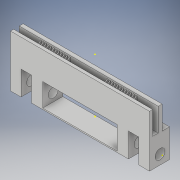
# Autodesk Inventor part: Xbelt Holder
Saved by Autodesk Inventor 2018 (Build 220112000, 112)
## iProperties
Created: 2018-02-26
Part Number: Xbelt Holder
Material: Generic
Document SubType Name: Modeling
Designer: junai
Density: 1 g/cm^3
Appearance: Default
Mass: 48.8128 g
Surface Area: 308.114 cm^2
Volume: 48.8128 cm^3
Author: junai
Autodesk Inventor part; units mm, degrees
ref_plane "YZ Plane" through (0, 0, 0) normal (1, 0, 0) x (0, 1, 0)
ref_plane "XZ Plane" through (0, 0, 0) normal (0, 1, 0) x (-1, 0, 0)
ref_plane "XY Plane" through (0, 0, 0) normal (0, 0, 1) x (1, 0, 0)
sketch "Sketch1" plane through (0, 0, 0) normal (0, 1, 0) x (-1, 0, 0)
  point P0 (0, 0)
sketch "Sketch2" plane through (0, 0, 0) normal (0, 1, 0) x (-1, 0, 0)
  line L0 (68.1059, 14.081) -> (-63.8941, 14.081)
  line L1 (-63.8941, 14.081) -> (-63.8941, -10.919)
  line L2 (-63.8941, -10.919) -> (68.1059, -10.919)
  line L3 (68.1059, -10.919) -> (68.1059, 14.081)
  point P0 (0, 0)
  dimension "d0" = 132
  dimension "d1" = 25
  constraints: 8 end point, 2 parallel, 1 horizontal, 1 perpendicular
  measures "d0" distance of L2.end L1.end
  measures "d1" distance of L0.end L1.end
extrude "Extrusion2" add sketch "Sketch2" along normal blind 6
sketch "Sketch4" plane through (0, 6, 0) normal (0, 1, 0) x (1, 0, 0)
  line L0 (-68.1059, -14.081) -> (63.8941, -14.081) projected
  line L1 (-68.1059, -14.081) -> (63.8941, -14.081)
  line L2 (63.8941, -14.081) -> (63.8941, -9.081)
  line L3 (63.8941, -9.081) -> (-68.1059, -9.081)
  line L4 (-68.1059, -9.081) -> (-68.1059, -14.081)
  line L5 (63.8941, -14.081) -> (63.8941, 10.919) projected
  point P0 (0, 0)
  dimension "d7" = 5
  constraints: 8 end point, 2 parallel, 1 collinear, 1 horizontal, 1 perpendicular
  measures "d7" distance of L1.end L2.end
extrude "Extrusion3" add sketch "Sketch4" along normal blind 45
sketch "Sketch5" plane through (0, 6, 0) normal (0, 1, 0) x (1, 0, 0)
  line L0 (63.8941, 10.919) -> (-68.1059, 10.919) projected
  line L1 (-68.1059, 10.919) -> (63.8941, 10.919)
  line L2 (63.8941, 10.919) -> (63.8941, -1.081)
  line L3 (63.8941, -1.081) -> (-68.1059, -1.081)
  line L4 (-68.1059, -1.081) -> (-68.1059, 10.919)
  line L5 (63.8941, -9.081) -> (63.8941, 10.919) projected
  point P0 (0, 0)
  dimension "d10" = 12
  constraints: 8 end point, 2 parallel, 1 collinear, 1 horizontal, 1 perpendicular
  measures "d10" distance of L1.end L2.end
extrude "Extrusion4" add sketch "Sketch5" along normal blind 45
sketch "Sketch6" plane through (0, 0, 0) normal (0, -1, 0) x (1, 0, 0)
  line L0 (63.8941, -10.919) -> (-68.1059, -10.919) projected
  line L1 (63.8941, -10.919) -> (-68.1059, -10.919)
  line L2 (-68.1059, -10.919) -> (-68.1059, -1.919)
  line L3 (-68.1059, -1.919) -> (63.8941, -1.919)
  line L4 (63.8941, -1.919) -> (63.8941, -10.919)
  line L5 (-68.1059, -10.919) -> (-68.1059, 14.081) projected
  point P0 (0, 0)
  dimension "d13" = 9
  constraints: 8 end point, 2 parallel, 1 collinear, 1 horizontal, 1 perpendicular
  measures "d13" distance of L1.end L2.end
extrude "Extrusion5" cut sketch "Sketch6" against normal blind 26
sketch "Sketch10" plane through (0, 51, 0) normal (0, 1, 0) x (1, 0, 0)
  point P0 (0, 0)
sketch "Sketch11" plane through (0, 51, 0) normal (0, 1, 0) x (1, 0, 0)
  line L0 (-58.1059, 1.919) -> (-48.1059, 1.919) construction
  line L1 (53.8941, 1.919) -> (43.8941, 1.919) construction
  line L2 (63.8941, 10.919) -> (-68.1059, 10.919) projected
  line L3 (-48.1059, 1.919) -> (-58.1059, 1.919)
  line L4 (-58.1059, 1.919) -> (-58.1059, 10.919)
  line L5 (-58.1059, 10.919) -> (-48.1059, 10.919)
  line L6 (-48.1059, 10.919) -> (-48.1059, 1.919)
  line L7 (43.8941, 1.919) -> (53.8941, 1.919)
  line L8 (53.8941, 1.919) -> (53.8941, 10.919)
  line L9 (53.8941, 10.919) -> (43.8941, 10.919)
  line L10 (43.8941, 10.919) -> (43.8941, 1.919)
  line L11 (-68.1059, -1.081) -> (-68.1059, -9.081) construction
  line L12 (-68.1059, -1.081) -> (-58.1059, -1.081) construction
  line L13 (-58.1059, -1.081) -> (-58.1059, 1.919) construction
  line L14 (63.8941, -1.081) -> (53.8941, -1.081) construction
  line L15 (-68.1059, -1.081) -> (63.8941, -1.081) construction
  line L16 (53.8941, -1.081) -> (53.8941, 1.919) construction
  point P0 (0, 0)
  dimension "d21" = 10
  dimension "d23" = 10
  dimension "d26" = 10
  dimension "d27" = 9
  dimension "d28" = 9
  dimension "d29" = 10
  dimension "d30" = 10
  constraints: 28 end point, 4 parallel, 4 perpendicular, 3 horizontal, 3 point on line
  measures "d21" distance of L0.start L0.end
  measures "d23" distance of L1.start L1.end
  measures "d26" distance between parallel lines of L6 L4
  measures "d27" distance of L9.end L1.end
  measures "d28" distance of L5.end L0.end
  measures "d29" distance of L11.start L12.end
  measures "d30" distance of L14.start L14.end
extrude "Extrusion6" cut sketch "Sketch11" against normal blind 26
sketch "Sketch13" plane through (0, 6, 0) normal (0, 1, 0) x (1, 0, 0)
  line L0 (-48.1059, 1.919) -> (-48.1059, -9.1654) construction
  line L1 (-48.1059, -1.081) -> (-47.0059, -1.081)
  constraints: 4 end point, 1 horizontal, 1 point on line, 1 vertical
sketch "Sketch14" plane through (0, 51, 0) normal (0, 1, 0) x (1, 0, 0)
  line L0 (-68.1059, -1.081) -> (-68.1059, -9.081) projected
  line L1 (-68.1059, -1.081) -> (63.8941, -1.081)
  line L2 (63.8941, -1.081) -> (63.8941, -4.081)
  line L3 (63.8941, -4.081) -> (-68.1059, -4.081)
  line L4 (-68.1059, -4.081) -> (-68.1059, -1.081)
  line L5 (63.8941, -9.081) -> (63.8941, -1.081) projected
  point P0 (0, 0)
  dimension "d35" = 3
  constraints: 8 end point, 2 parallel, 1 collinear, 1 horizontal, 1 perpendicular
  measures "d35" distance of L1.end L2.end
extrude "Extrusion7" add sketch "Sketch14" against normal up to next
sketch "Sketch15" plane through (0, 51, 0) normal (0, 1, 0) x (1, 0, 0)
  line L0 (-68.1059, 1.919) -> (63.8941, 1.919) projected
  line L1 (-58.3742, 1.919) -> (-48.1059, 1.919)
  line L2 (-48.1059, 1.919) -> (-48.1059, -0.081)
  line L3 (-48.1059, -0.081) -> (-58.3742, -0.081)
  line L4 (-58.3742, -0.081) -> (-58.3742, 1.919)
  line L5 (-48.1059, 10.919) -> (-48.1059, 1.919) projected
  line L6 (53.8941, 1.919) -> (43.8941, 1.919) projected
  line L7 (43.8941, 1.919) -> (53.8941, 1.919)
  line L8 (53.8941, 1.919) -> (53.8941, -0.081)
  line L9 (53.8941, -0.081) -> (43.8941, -0.081)
  line L10 (43.8941, -0.081) -> (43.8941, 1.919)
  line L11 (53.8941, 10.919) -> (53.8941, 1.919) projected
  point P0 (0, 0)
  dimension "d38" = 2
  dimension "d39" = 2
  constraints: 16 end point, 4 parallel, 2 collinear, 2 horizontal, 2 perpendicular, 1 point on line
  measures "d38" distance of L1.end L2.end
  measures "d39" distance of L7.end L8.end
extrude "Extrusion8" cut sketch "Sketch15" against normal up to next
sketch "Sketch16" plane through (0, 0, 0) normal (0, -1, 0) x (1, 0, 0)
  line L0 (53.8941, -1.919) -> (63.8941, -1.919) projected
  line L1 (63.8941, -1.919) -> (-68.1059, -1.919)
  line L2 (-68.1059, -1.919) -> (-68.1059, 0.081)
  line L3 (-68.1059, 0.081) -> (63.8941, 0.081)
  line L4 (63.8941, 0.081) -> (63.8941, -1.919)
  line L5 (-68.1059, -1.919) -> (-68.1059, 14.081) projected
  point P0 (0, 0)
  dimension "d42" = 2
  constraints: 8 end point, 2 parallel, 1 collinear, 1 horizontal, 1 perpendicular
  measures "d42" distance of L1.end L2.end
extrude "Extrusion9" cut sketch "Sketch16" against normal up to surface (26 mm away)
sketch "Sketch17" plane through (0, 6, 0) normal (0, 1, 0) x (1, 0, 0)
  point P0 (0, 0)
sketch "Sketch18" plane through (0, 51, 0) normal (0, 1, 0) x (1, 0, 0)
  line L0 (-58.3742, 1.919) -> (-58.1059, 1.919) projected
  line L1 (-48.1059, -0.081) -> (-58.3742, -0.081) projected
  line L2 (-58.1059, 1.919) -> (-58.3742, 1.919)
  line L3 (-58.3742, 1.919) -> (-58.3742, -0.081)
  line L4 (-58.3742, -0.081) -> (-58.1059, -0.081)
  line L5 (-58.1059, -0.081) -> (-58.1059, 1.919)
  point P0 (0, 0)
  constraints: 8 end point, 2 parallel, 1 horizontal, 1 perpendicular
extrude "Extrusion10" add sketch "Sketch18" against normal blind 25
sketch "Sketch19" plane through (0, 6, 0) normal (0, 1, 0) x (1, 0, 0)
  line L0 (-48.1059, 10.919) -> (-48.1059, -0.081) construction
  line L1 (-48.1059, -0.081) -> (-48.1059, -9.081) construction
  line L2 (63.8941, -9.081) -> (-68.1059, -9.081) construction
  line L3 (63.8941, -4.081) -> (-68.1059, -4.081) projected
  line L4 (-48.1059, -4.081) -> (-47.0059, -4.081)
  line L5 (-47.0059, -4.081) -> (-47.0059, -8.481)
  line L6 (-47.0059, -8.481) -> (-48.1059, -8.481)
  line L7 (-48.1059, -8.481) -> (-48.1059, -4.081)
  line L8 (-48.1059, -9.081) -> (-48.1059, -8.481) construction
  point P0 (0, 0)
  dimension "d47" = 1.1
  dimension "d49" = 0.6
  constraints: 12 end point, 4 point on line, 2 parallel, 1 horizontal, 1 perpendicular, 1 vertical
  measures "d47" distance of L6.end L5.end
  measures "d49" distance of L1.end L6.end
extrude "Extrusion11" add sketch "Sketch19" along normal blind 45
sketch "Sketch20" plane through (0, 6, 0) normal (0, 1, 0) x (1, 0, 0)
  line L0 (63.8941, -9.081) -> (-68.1059, -9.081) projected
  line L1 (63.8941, -4.081) -> (-47.0059, -4.081) projected
  line L2 (-68.1059, -9.081) -> (63.8941, -9.081)
  line L3 (63.8941, -9.081) -> (63.8941, -4.081)
  line L4 (63.8941, -4.081) -> (-68.1059, -4.081)
  line L5 (-68.1059, -4.081) -> (-68.1059, -9.081)
  point P0 (0, 0)
  constraints: 8 end point, 2 parallel, 1 horizontal, 1 perpendicular
extrude "Extrusion12" add sketch "Sketch20" along normal blind 6
sketch "Sketch21" plane through (0, 0, 0) normal (0, -1, 0) x (1, 0, 0)
  line L0 (63.8941, 14.081) -> (63.8941, 0.081) projected
  line L1 (-68.1059, -10.919) -> (-68.1059, 0.081) projected
  line L2 (63.8941, 14.081) -> (-68.1059, 14.081)
  line L3 (-68.1059, 14.081) -> (-68.1059, 0.081)
  line L4 (-68.1059, 0.081) -> (63.8941, 0.081)
  line L5 (63.8941, 0.081) -> (63.8941, 14.081)
  point P0 (0, 0)
  constraints: 8 end point, 2 parallel, 1 horizontal, 1 perpendicular
extrude "Extrusion13" cut sketch "Sketch21" against normal blind 6
sketch "Sketch22" plane through (0, 51, 0) normal (0, 1, 0) x (1, 0, 0)
  line L0 (-48.1059, -8.481) -> (-47.0059, -8.481) projected
  line L1 (63.8941, -4.081) -> (-47.0059, -4.081) projected
  line L2 (-48.1059, -8.481) -> (-47.0059, -8.481)
  line L3 (-47.0059, -8.481) -> (-47.0059, -4.081)
  line L4 (-47.0059, -4.081) -> (-48.1059, -4.081)
  line L5 (-48.1059, -4.081) -> (-48.1059, -8.481)
  point P0 (0, 0)
  constraints: 8 end point, 2 parallel, 1 horizontal, 1 perpendicular
extrude "Extrusion14" cut sketch "Sketch22" against normal blind 1
sketch "Sketch23" plane through (-47.0059, 12, 8.481) normal (1, 0, 0) x (0, 0, -1)
  point P0 (8.481, -12)
pattern_linear "Rectangular Pattern3" count 8 spacing 2.5 along (1, 0, 0) of "Extrusion11"
sketch "Sketch24" plane through (0, 51, 0) normal (0, 1, 0) x (1, 0, 0)
  line L0 (-45.6059, -4.081) -> (-45.6059, -8.481) projected
  line L1 (-44.5059, -4.081) -> (-43.1059, -4.081) projected
  line L2 (-45.6059, -8.481) -> (-44.5059, -8.481)
  line L3 (-44.5059, -8.481) -> (-44.5059, -4.081)
  line L4 (-44.5059, -4.081) -> (-45.6059, -4.081)
  line L5 (-45.6059, -4.081) -> (-45.6059, -8.481)
  line L6 (-43.1059, -8.481) -> (-42.0059, -8.481) projected
  line L7 (-40.6059, -4.081) -> (-42.0059, -4.081) projected
  line L8 (-43.1059, -8.481) -> (-42.0059, -8.481)
  line L9 (-42.0059, -8.481) -> (-42.0059, -4.081)
  line L10 (-42.0059, -4.081) -> (-43.1059, -4.081)
  line L11 (-43.1059, -4.081) -> (-43.1059, -8.481)
  line L12 (-38.1059, -4.081) -> (-39.5059, -4.081) projected
  line L13 (-40.6059, -4.081) -> (-40.6059, -8.481) projected
  line L14 (-39.5059, -4.081) -> (-40.6059, -4.081)
  line L15 (-40.6059, -4.081) -> (-40.6059, -8.481)
  line L16 (-40.6059, -8.481) -> (-39.5059, -8.481)
  line L17 (-39.5059, -8.481) -> (-39.5059, -4.081)
  line L18 (-35.6059, -4.081) -> (-37.0059, -4.081) projected
  line L19 (-38.1059, -4.081) -> (-38.1059, -8.481) projected
  line L20 (-37.0059, -4.081) -> (-38.1059, -4.081)
  line L21 (-38.1059, -4.081) -> (-38.1059, -8.481)
  line L22 (-38.1059, -8.481) -> (-37.0059, -8.481)
  line L23 (-37.0059, -8.481) -> (-37.0059, -4.081)
  line L24 (-33.1059, -4.081) -> (-34.5059, -4.081) projected
  line L25 (-35.6059, -4.081) -> (-35.6059, -8.481) projected
  line L26 (-34.5059, -4.081) -> (-35.6059, -4.081)
  line L27 (-35.6059, -4.081) -> (-35.6059, -8.481)
  line L28 (-35.6059, -8.481) -> (-34.5059, -8.481)
  line L29 (-34.5059, -8.481) -> (-34.5059, -4.081)
  line L30 (-30.6059, -4.081) -> (-32.0059, -4.081) projected
  line L31 (-33.1059, -8.481) -> (-33.1059, -4.081) projected
  line L32 (-32.0059, -4.081) -> (-33.1059, -4.081)
  line L33 (-33.1059, -4.081) -> (-33.1059, -8.481)
  line L34 (-33.1059, -8.481) -> (-32.0059, -8.481)
  line L35 (-32.0059, -8.481) -> (-32.0059, -4.081)
  line L36 (-29.5059, -4.081) -> (-29.5059, -8.481) projected
  line L37 (-29.5059, -8.481) -> (-30.6059, -8.481) projected
  line L38 (-29.5059, -4.081) -> (-30.6059, -4.081)
  line L39 (-30.6059, -4.081) -> (-30.6059, -8.481)
  line L40 (-30.6059, -8.481) -> (-29.5059, -8.481)
  line L41 (-29.5059, -8.481) -> (-29.5059, -4.081)
  point P0 (0, 0)
  constraints: 56 end point, 14 parallel, 7 horizontal, 7 perpendicular
extrude "Extrusion15" cut sketch "Sketch24" against normal blind 1
draft "FaceDraft1" angle 12.8 pull direction (0, 0, 1) faces at (-47.3726, 50, 7.0143) fixed edges at (-47.5559, 50, 8.481)
draft "FaceDraft2" angle 12.8 pull direction (0, 0, 1) faces at (-45.2392, 50, 5.5476) fixed edges at (-45.0559, 50, 8.481)
draft "FaceDraft3" angle 12.8 pull direction (0, 0, 1) faces at (-42.7392, 50, 5.5476) (-40.2392, 50, 5.5476) (-37.7392, 50, 5.5476) fixed edges at (-42.5559, 50, 8.481) (-40.0559, 50, 8.481) (-37.5559, 50, 8.481)
draft "FaceDraft4" angle 12.8 pull direction (0, 0, 1) faces at (-35.2392, 50, 5.5476) (-32.7392, 50, 5.5476) (-30.2392, 50, 5.5476) fixed edges at (-35.0559, 50, 8.481) (-32.5559, 50, 8.481) (-30.0559, 50, 8.481)
pattern_linear "Rectangular Pattern4" count 2 spacing 73.5 along (1, 0, 0) of "Extrusion15", "Extrusion14"
sketch "Sketch25" plane through (0, 51, 0) normal (0, 1, 0) x (1, 0, 0)
  line L0 (43.8941, -0.081) -> (43.8941, 10.919) construction
  line L1 (43.8941, -0.081) -> (43.8941, -9.0359) construction
  line L2 (63.8941, -4.081) -> (-68.1059, -4.081) projected
  line L3 (43.8941, -4.081) -> (42.7941, -4.081)
  line L4 (42.7941, -4.081) -> (42.7941, -8.481)
  line L5 (42.7941, -8.481) -> (43.8941, -8.481)
  line L6 (43.8941, -8.481) -> (43.8941, -4.081)
  point P0 (0, 0)
  dimension "d76" = 1.1
  dimension "d77" = 4.4
  constraints: 10 end point, 2 parallel, 2 point on line, 1 horizontal, 1 perpendicular, 1 vertical
  measures "d76" distance of L5.end L4.end
  measures "d77" distance of L3.end L4.end
extrude "Extrusion16" add sketch "Sketch25" against normal up to next
sketch "Sketch26" plane through (0, 51, 0) normal (0, 1, 0) x (1, 0, 0)
  line L0 (42.7941, -8.481) -> (42.7941, -4.081) projected
  line L1 (63.8941, -4.081) -> (43.8941, -4.081) projected
  line L2 (42.7941, -8.481) -> (43.8941, -8.481)
  line L3 (43.8941, -8.481) -> (43.8941, -4.081)
  line L4 (43.8941, -4.081) -> (42.7941, -4.081)
  line L5 (42.7941, -4.081) -> (42.7941, -8.481)
  point P0 (0, 0)
  constraints: 8 end point, 2 parallel, 1 horizontal, 1 perpendicular
extrude "Extrusion17" cut sketch "Sketch26" against normal blind 1
pattern_linear "Rectangular Pattern5" count 8 spacing 2.5 along (-1, 0, 0) of "Extrusion16", "Extrusion17"
draft "FaceDraft5" angle 12.8 pull direction (0, 0, 1) faces at (43.1608, 50, 5.5476) (40.6608, 50, 5.5476) (38.1608, 50, 5.5476) (35.6608, 50, 5.5476) fixed edges at (43.3441, 50, 8.481) (40.8441, 50, 8.481) (38.3441, 50, 8.481) (35.8441, 50, 8.481)
draft "FaceDraft6" angle 12.8 pull direction (0, 0, 1) faces at (33.1608, 50, 5.5476) (30.6608, 50, 5.5476) (28.1608, 50, 5.5476) (25.6608, 50, 5.5476) fixed edges at (33.3441, 50, 8.481) (30.8441, 50, 8.481) (28.3441, 50, 8.481) (25.8441, 50, 8.481)
sketch "Sketch27" plane through (63.8941, 51, 14.081) normal (1, 0, 0) x (0, 0, -1)
  point P0 (14.081, -51)
sketch "Sketch29" plane through (63.8941, 51, 14.081) normal (1, 0, 0) x (0, 0, -1)
  point P0 (14.081, -51)
sketch "Sketch32" plane through (-68.1059, 51, 9.081) normal (-1, 0, 0) x (0, 0, 1)
  point P0 (-9.081, -51)
sketch "Sketch33" plane through (-68.1059, 51, 9.081) normal (-1, 0, 0) x (0, 0, 1)
  line L0 (-20, 0) -> (-20, -25) projected
  line L1 (-20, -25) -> (-24.35, -25)
  line L2 (-24.35, -25) -> (-24.35, 0)
  line L3 (-24.35, 0) -> (-20, 0)
  line L4 (-20, 0) -> (-20, -25)
  line L5 (-20, 0) -> (-5, 0) projected
  line L6 (-20, -25) -> (-24.35, -25) construction
  point P0 (-9.081, -51)
  dimension "d96" = 4.35
  dimension "d97" = 25
  dimension "d98" = 4.35
  constraints: 10 end point, 2 horizontal, 2 parallel, 1 collinear, 1 perpendicular
  measures "d96" distance of L2.end L3.end
  measures "d97" distance of L0.start L0.end
  measures "d98" distance of L0.end L1.end
sketch "Sketch34" plane through (63.8941, 51, 14.081) normal (1, 0, 0) x (0, 0, -1)
  line L0 (0, -45) -> (0, 0) projected
  line L1 (14, -25) -> (14, -45) projected
  line L2 (0, -45) -> (14, -45)
  line L3 (14, -45) -> (14, -25)
  line L4 (14, -25) -> (0, -25)
  line L5 (0, -25) -> (0, -45)
  point P0 (14.081, -51)
  constraints: 8 end point, 2 parallel, 1 horizontal, 1 perpendicular
extrude "Extrusion20" add sketch "Sketch33" against normal blind 132
extrude "Extrusion21" add sketch "Sketch34" against normal blind 132
sketch "Sketch35" plane through (63.8941, 51, 14.081) normal (1, 0, 0) x (0, 0, -1)
  line L0 (14, -45) -> (14, -25) projected
  line L1 (14, -45) -> (0, -45)
  line L2 (0, -45) -> (0, -30.9976)
  line L3 (0, -30.9976) -> (14, -30.9976)
  line L4 (14, -30.9976) -> (14, -45)
  line L5 (5.184, -24.9976) -> (5.184, -30.9976) construction
  line L6 (0, -45) -> (0, 0) construction
  point P0 (14.081, -51)
  dimension "d103" = 6
  constraints: 10 end point, 2 parallel, 2 perpendicular, 1 collinear, 1 horizontal, 1 point on line
  measures "d103" distance of L5.start L5.end
extrude "Extrusion22" cut sketch "Sketch35" against normal blind 132
sketch "Sketch36" plane through (0, 51, 0) normal (0, 1, 0) x (1, 0, 0)
  line L0 (43.8941, 10.919) -> (53.8941, 10.919) projected
  line L1 (-68.1059, 15.269) -> (63.8941, 15.269) projected
  line L2 (43.8941, 10.919) -> (53.8941, 10.919)
  line L3 (53.8941, 10.919) -> (53.8941, 15.269)
  line L4 (53.8941, 15.269) -> (43.8941, 15.269)
  line L5 (43.8941, 15.269) -> (43.8941, 10.919)
  line L6 (53.8941, 10.919) -> (53.8941, -0.081) projected
  point P0 (0, 0)
  constraints: 8 end point, 2 parallel, 1 collinear, 1 horizontal, 1 perpendicular, 1 point on line
sketch "Sketch37" plane through (0, 51, 0) normal (0, 1, 0) x (1, 0, 0)
  line L0 (-48.1059, -0.081) -> (-48.1059, 10.919) projected
  line L1 (-68.1059, 15.269) -> (63.8941, 15.269) projected
  line L2 (-48.1059, 10.919) -> (-58.1059, 10.919)
  line L3 (-58.1059, 10.919) -> (-58.1059, 15.269)
  line L4 (-58.1059, 15.269) -> (-48.1059, 15.269)
  line L5 (-48.1059, 15.269) -> (-48.1059, 10.919)
  line L6 (-58.1059, -0.081) -> (-58.1059, 10.919) projected
  point P0 (0, 0)
  constraints: 8 end point, 2 parallel, 1 collinear, 1 horizontal, 1 perpendicular, 1 point on line
extrude "Extrusion23" cut sketch "Sketch37" against normal through all
extrude "Extrusion24" cut sketch "Sketch36" against normal blind 132
sketch "Sketch38" plane through (-68.1059, 51, 9.081) normal (-1, 0, 0) x (0, 0, 1)
  circle A0 centre (-19.85, -12.5) radius 4.5
  line L0 (-24.35, -25) -> (-24.35, 0) projected
  point P0 (-9.081, -51)
  point P1 (-24.35, -12.5)
  dimension "d111" = 9
  constraints: 1 horizontal alignment, 1 midpoint, 1 vertical, 2 other
extrude "Extrusion25" cut sketch "Sketch38" against normal blind 132
sketch "Sketch39" plane through (0, 51, 0) normal (0, 1, 0) x (1, 0, 0)
  line L0 (63.8941, -4.081) -> (-68.1059, -4.081) construction
  line L1 (63.8941, -0.081) -> (-68.1059, -0.081) construction
  line L2 (25.2951, -4.081) -> (-29.5059, -4.081) construction
  line L3 (-29.5059, -4.081) -> (-29.5059, -0.081) construction
  line L4 (-29.5059, -0.081) -> (25.2951, -0.081) construction
  line L5 (25.2951, -0.081) -> (25.2951, -4.081) construction
  line L6 (-29.5059, -4.081) -> (-29.5059, -8.481) construction
  line L7 (-48.1059, 15.269) -> (43.8941, 15.269) projected
  line L8 (-29.5059, -0.081) -> (25.2951, -0.081)
  line L9 (25.2951, -0.081) -> (25.2951, 15.269)
  line L10 (25.2951, 15.269) -> (-29.5059, 15.269)
  line L11 (-29.5059, 15.269) -> (-29.5059, -0.081)
  point P0 (0, 0)
  constraints: 16 end point, 4 parallel, 3 point on line, 2 collinear, 2 horizontal, 2 perpendicular
extrude "Extrusion26" cut sketch "Sketch39" against normal blind 132
sketch "Sketch40" plane through (-68.1059, 51, 9.081) normal (-1, 0, 0) x (0, 0, 1)
  line L0 (-9, -25) -> (-24.35, -25) projected
  line L1 (-24.35, -25) -> (-25.817, -25)
  line L2 (-25.817, -25) -> (-25.817, 0)
  line L3 (-25.817, 0) -> (-24.35, 0)
  line L4 (-24.35, 0) -> (-24.35, -25)
  line L5 (-24.35, 0) -> (-5, 0) projected
  point P0 (-9.081, -51)
  dimension "d116" = 1.467
  constraints: 8 end point, 2 parallel, 1 collinear, 1 horizontal, 1 perpendicular
extrude "Extrusion27" add sketch "Sketch40" against normal blind 132
pattern_linear "Rectangular Pattern6" count 5 spacing 2.5 along (-1, 0, 0) of "Extrusion14", "Extrusion11"
pattern_linear "Rectangular Pattern7" count 5 spacing 2.5 along (1, 0, 0) of "Extrusion17", "Extrusion16"
draft "FaceDraft7" angle 12.8 pull direction (0, 0, 1) faces at (53.1608, 50, 5.5476) (50.6608, 50, 5.5476) (48.1608, 50, 5.5476) (45.6608, 50, 5.5476) fixed edges at (53.3441, 50, 8.481) (50.8441, 50, 8.481) (48.3441, 50, 8.481) (45.8441, 50, 8.481)
draft "FaceDraft8" angle 12.8 pull direction (0, 0, 1) faces at (-49.8726, 50, 7.0143) (-52.3726, 50, 7.0143) (-54.8726, 50, 7.0143) (-57.3726, 50, 7.0143) fixed edges at (-50.0559, 50, 8.481) (-52.5559, 50, 8.481) (-55.0559, 50, 8.481) (-57.5559, 50, 8.481)
sketch "Sketch41" plane through (63.8941, 51, 14.081) normal (1, 0, 0) x (0, 0, -1)
  circle A0 centre (22.9612, -12.5) radius 4.5
  point P0 (14.081, -51)
  dimension "d127" = 9
  constraints: 1 centre point
  measures "d127" diameter of A0
sketch "Sketch42" plane through (63.8941, 51, 14.081) normal (1, 0, 0) x (0, 0, -1)
  point P0 (14.081, -51)
sketch "Sketch43" plane through (63.8941, 51, 14.081) normal (1, 0, 0) x (0, 0, -1)
  circle A0 centre (24.85, -12.5) radius 4.5
  circle A1 centre (24.85, -12.5) radius 4.5 projected
  point P0 (14.081, -51)
  dimension "d128" = 9
  constraints: 1 centre point, 1 concentric
  measures "d128" diameter of A0
extrude "Extrusion28" add sketch "Sketch43" against normal blind 132
extrude "Extrusion29" cut sketch "Sketch41" against normal blind 132
sketch "Sketch44" plane through (0, 51, 0) normal (0, 1, 0) x (1, 0, 0)
  line L0 (-58.1059, 15.269) -> (-48.1059, 15.269) projected
  line L1 (63.8941, -0.081) -> (-68.1059, -0.081) projected
  line L2 (-58.1059, 15.269) -> (-48.1059, 15.269)
  line L3 (-48.1059, 15.269) -> (-48.1059, -0.081)
  line L4 (-48.1059, -0.081) -> (-58.1059, -0.081)
  line L5 (-58.1059, -0.081) -> (-58.1059, 15.269)
  line L6 (-29.5059, 15.269) -> (25.2951, 15.269)
  line L7 (25.2951, 15.269) -> (25.2951, -0.081)
  line L8 (25.2951, -0.081) -> (-29.5059, -0.081)
  line L9 (-29.5059, -0.081) -> (-29.5059, 15.269)
  line L10 (43.8941, 15.269) -> (53.7113, 15.269)
  line L11 (53.7113, 15.269) -> (53.7113, -0.081)
  line L12 (53.7113, -0.081) -> (43.8941, -0.081)
  line L13 (43.8941, -0.081) -> (43.8941, 15.269)
  line L14 (-48.1059, 15.269) -> (-48.1059, -0.081) projected
  line L15 (-29.5059, -0.081) -> (-29.5059, 15.269) projected
  line L16 (25.2951, 15.269) -> (25.2951, -0.081) projected
  line L17 (43.8941, -0.081) -> (43.8941, 15.269) projected
  point P0 (0, 0)
  constraints: 24 end point, 6 parallel, 4 collinear, 3 horizontal, 3 perpendicular, 2 point on line, 4 other
extrude "Extrusion30" cut sketch "Sketch44" against normal blind 132
sketch "Sketch45" plane through (-68.1059, 51, 9.081) normal (-1, 0, 0) x (0, 0, 1)
  line L0 (-9, -30.9976) -> (-9, -25) projected
  line L1 (-9, -30.9976) -> (5, -30.9976)
  line L2 (5, -30.9976) -> (5, -46.0708)
  line L3 (5, -46.0708) -> (-9, -46.0708)
  line L4 (-9, -46.0708) -> (-9, -30.9976)
  line L5 (5, -30.9976) -> (5, 0) projected
  point P0 (-9.081, -51)
  constraints: 8 end point, 2 parallel, 1 collinear, 1 horizontal, 1 perpendicular
extrude "Extrusion31" cut sketch "Sketch45" against normal blind 132
sketch "Sketch46" plane through (0, 51, 0) normal (0, 1, 0) x (1, 0, 0)
  point P0 (0, 0)
sketch "Sketch47" plane through (63.8941, 26, 9.081) normal (0, 1, 0) x (1, 0, 0)
  point P0 (-63.8941, 9.081)
sketch "Sketch48" plane through (63.8941, 26, 9.081) normal (0, 1, 0) x (1, 0, 0)
  line L0 (-10, 5) -> (-10, 0.6) projected
  line L1 (0, 0) -> (-132, 0) projected
  line L2 (-10, 5) -> (-122, 5)
  line L3 (-122, 5) -> (-122, 0)
  line L4 (-122, 0) -> (-10, 0)
  line L5 (-10, 0) -> (-10, 5)
  line L6 (-122, 0.6) -> (-122, 5) projected
  point P0 (-63.8941, 9.081)
  constraints: 8 end point, 2 parallel, 1 collinear, 1 horizontal, 1 perpendicular, 1 point on line
extrude "Extrusion32" cut sketch "Sketch48" along normal blind 132
sketch "Sketch49" plane through (63.8941, 26, 9.081) normal (0, 1, 0) x (1, 0, 0)
  line L0 (-112, 24.35) -> (-112, 9) construction
  line L1 (-112, 9) -> (-112, 0) construction
  line L2 (0, 0) -> (-132, 0) construction
  line L3 (-112, 0) -> (-110.9, 0)
  line L4 (-110.9, 0) -> (-110.9, 4.4)
  line L5 (-110.9, 4.4) -> (-112, 4.4)
  line L6 (-112, 4.4) -> (-112, 0)
  line L7 (0, 5) -> (-132, 5) construction
  line L8 (-112, 5) -> (-112, 4.4) construction
  point P0 (-63.8941, 9.081)
  dimension "d139" = 1.1
  dimension "d140" = 0.6
  constraints: 12 end point, 4 point on line, 2 parallel, 1 horizontal, 1 perpendicular, 1 vertical
  measures "d139" distance of L5.end L4.end
  measures "d140" distance of L8.start L5.end
extrude "Extrusion33" add sketch "Sketch49" along normal blind 19
pattern_linear "Rectangular Pattern8" count 12 spacing 2.5 along (1, 0, 0) of "Extrusion33"
sketch "Sketch50" plane through (63.8941, 26, 9.081) normal (0, 1, 0) x (1, 0, 0)
  line L0 (-20, 24.35) -> (-20, 9) construction
  line L1 (-20, 9) -> (-20, 0) construction
  line L2 (-20, 5.0016) -> (-20, 4.4016) construction
  line L3 (0, 0) -> (-132, 0) projected
  line L4 (-20, 0) -> (-21.1, 0)
  line L5 (-21.1, 0) -> (-21.1, 4.4)
  line L6 (-21.1, 4.4) -> (-20, 4.4)
  line L7 (-20, 4.4) -> (-20, 0)
  point P0 (-63.8941, 9.081)
  dimension "d146" = 0.6
  dimension "d147" = 1.1
  dimension "d148" = 4.4
  constraints: 12 end point, 3 point on line, 2 parallel, 1 horizontal, 1 perpendicular, 1 vertical
  measures "d146" distance of L2.start L2.end
  measures "d147" distance of L5.end L6.end
  measures "d148" distance of L4.end L5.end
extrude "Extrusion34" add sketch "Sketch50" along normal blind 19
pattern_linear "Rectangular Pattern9" count 12 spacing 2.5 along (-1, 0, 0) of "Extrusion34"
draft "FaceDraft9" angle 50 pull direction (0, 0, -1) faces at (43.5274, 45, 7.6143) (41.0274, 45, 7.6143) (38.5274, 45, 7.6143) (36.0274, 45, 7.6143) (33.5274, 45, 6.1476) (31.0274, 45, 6.1476) (28.5274, 45, 7.6143) (26.0274, 45, 7.6143) (23.5274, 45, 7.6143) (21.0274, 45, 7.6143) (18.5274, 45, 7.6143) (16.0274, 45, 6.1476) fixed edges at (43.3441, 45, 4.681) (40.8441, 45, 4.681) (38.3441, 45, 4.681) (35.8441, 45, 4.681) (33.3441, 45, 4.681) (30.8441, 45, 4.681) (28.3441, 45, 4.681) (25.8441, 45, 4.681) (23.3441, 45, 4.681) (20.8441, 45, 4.681) (18.3441, 45, 4.681) (15.8441, 45, 4.681)
draft "FaceDraft10" angle 50 pull direction (0, 0, -1) faces at (-19.8726, 45, 6.1476) (-22.3726, 45, 6.1476) (-24.8726, 45, 6.1476) (-27.3726, 45, 6.1476) (-29.8726, 45, 6.1476) (-32.3726, 45, 6.1476) (-34.8726, 45, 6.1476) (-37.3726, 45, 6.1476) (-39.8726, 45, 6.1476) (-42.3726, 45, 6.1476) (-44.8726, 45, 6.1476) (-47.3726, 45, 7.6143) fixed edges at (-20.0559, 45, 4.681) (-22.5559, 45, 4.681) (-25.0559, 45, 4.681) (-27.5559, 45, 4.681) (-30.0559, 45, 4.681) (-32.5559, 45, 4.681) (-35.0559, 45, 4.681) (-37.5559, 45, 4.681) (-40.0559, 45, 4.681) (-42.5559, 45, 4.681) (-45.0559, 45, 4.681) (-47.5559, 45, 4.681)
sketch "Sketch51" plane through (0, 51, 0) normal (0, 1, 0) x (1, 0, 0)
  line L0 (53.8941, 9.8246) -> (53.8941, 15.269) projected
  line L1 (53.8941, 15.269) -> (49.2702, 15.269)
  line L2 (49.2702, 15.269) -> (49.2702, 6.1586)
  line L3 (49.2702, 6.1586) -> (53.8941, 6.1586)
  line L4 (53.8941, 6.1586) -> (53.8941, 15.269)
  point P0 (0, 0)
  constraints: 8 end point, 2 parallel, 1 horizontal, 1 perpendicular
extrude "Extrusion35" cut sketch "Sketch51" against normal blind 20
sketch "Sketch52" plane through (63.8941, 51, 14.081) normal (1, 0, 0) x (0, 0, -1)
  line L0 (14, -25) -> (29.35, -25) projected
  line L1 (30.817, 0) -> (10, 0) projected
  line L2 (14, -25) -> (30.817, -25)
  line L3 (30.817, -25) -> (30.817, 0)
  line L4 (30.817, 0) -> (14, 0)
  line L5 (14, 0) -> (14, -25)
  point P0 (14.081, -51)
  constraints: 8 end point, 2 parallel, 1 horizontal, 1 perpendicular
extrude "Extrusion36" cut sketch "Sketch52" against normal through all
sketch "Sketch53" plane through (63.8941, 51, 14.081) normal (1, 0, 0) x (0, 0, -1)
  line L0 (0, -30.9976) -> (0, 0) projected
  line L1 (0, 0) -> (2, 0)
  line L2 (2, 0) -> (2, -30.9976)
  line L3 (2, -30.9976) -> (0, -30.9976)
  line L4 (0, -30.9976) -> (0, 0)
  line L5 (0, -30.9976) -> (14, -30.9976) projected
  point P0 (14.081, -51)
  dimension "d160" = 2
  constraints: 8 end point, 2 parallel, 1 collinear, 1 horizontal, 1 perpendicular
  measures "d160" distance of L2.end L3.end
extrude "Extrusion37" cut sketch "Sketch53" against normal through all
sketch "Sketch54" plane through (-68.1059, 51, 0.081) normal (-1, 0, 0) x (0, 0, 1)
  point P0 (-0.081, -51)
sketch "Sketch55" plane through (-68.1059, 51, 0.081) normal (-1, 0, 0) x (0, 0, 1)
  point P0 (-0.081, -51)
sketch "Sketch56" plane through (-68.1059, 51, 0.081) normal (-1, 0, 0) x (0, 0, 1)
  line L0 (12, -30.9976) -> (0, -30.9976) projected
  line L1 (12, -30.9976) -> (-13, -30.9976)
  line L2 (-13, -30.9976) -> (-13, -51.8076)
  line L3 (-13, -51.8076) -> (12, -51.8076)
  line L4 (12, -51.8076) -> (12, -30.9976)
  point P0 (-0.081, -51)
  dimension "d163" = 20.81
  dimension "d164" = 25
  constraints: 8 end point, 2 parallel, 1 horizontal, 1 perpendicular
  measures "d163" distance of L1.end L2.end
  measures "d164" distance of L2.end L3.end
extrude "Extrusion38" add sketch "Sketch56" against normal blind 132
sketch "Sketch57" plane through (-68.1059, 51, 0.081) normal (-1, 0, 0) x (0, 0, 1)
  point P0 (-0.081, -51)
sketch "Sketch58" plane through (-68.1059, 51, 0.081) normal (-1, 0, 0) x (0, 0, 1)
  line L0 (-13, -51.8076) -> (12, -51.8076) construction
  line L1 (12, 0) -> (12, -51.8076) construction
  line L2 (12, -43.9516) -> (5, -43.9516) construction
  circle A0 centre (5, -43.9516) radius 4.5
  point P0 (-0.081, -51)
  dimension "d190" = 9
  dimension "d191" = 7
  constraints: 2 end point, 1 centre point, 1 coincident, 1 horizontal, 1 point on line
  measures "d190" diameter of A0
  measures "d191" distance of L2.start L2.end
sketch "Sketch59" plane through (-68.1059, -0.8076, -12.919) normal (0, 0, -1) x (-1, 0, 0)
  line L0 (0, 20.81) -> (0, 0) construction
  line L1 (-10, 16.81) -> (-20, 16.81)
  line L2 (-20, 16.81) -> (-20, 0)
  line L3 (-20, 0) -> (-10, 0)
  line L4 (-10, 0) -> (-10, 16.81)
  line L5 (0, 20.81) -> (-132, 20.81) projected
  line L6 (-132, 0) -> (-132, 20.81) construction
  line L7 (-132, 10.405) -> (-122, 10.405) construction
  line L8 (0, 0) -> (-132, 0) projected
  line L9 (-122, 0) -> (-112, 0)
  line L10 (-112, 0) -> (-112, 16.81)
  line L11 (-112, 16.81) -> (-122, 16.81)
  line L12 (-122, 16.81) -> (-122, 0)
  line L13 (-38.6, 16.81) -> (-93.4, 16.81)
  line L14 (-93.4, 16.81) -> (-93.4, 2)
  line L15 (-93.4, 2) -> (-38.6, 2)
  line L16 (-38.6, 2) -> (-38.6, 16.81)
  line L17 (-66, 0) -> (-66, 2) construction
  point P0 (-68.1059, 0.8076)
  dimension "d172" = 10
  dimension "d173" = 10
  dimension "d175" = 4
  dimension "d176" = 10
  dimension "d177" = 10
  dimension "d178" = 4
  dimension "d179" = 10
  dimension "d183" = 2
  dimension "d184" = 18.6
  dimension "d185" = 4
  dimension "d186" = 16.81
  dimension "d187" = 16.81
  constraints: 28 end point, 6 parallel, 4 horizontal, 3 midpoint, 3 perpendicular, 1 point on line, 1 vertical
  measures "d172" distance of L3.end L2.end
  measures "d173" distance between parallel lines of L4 L0
  measures "d175" distance between parallel lines of L5 L1
  measures "d176" distance of L7.start L7.end
  measures "d177" distance of L9.start L9.end
  measures "d178" distance between parallel lines of L5 L11
  measures "d179" distance between parallel lines of L6 L12
  measures "d183" distance of L17.end L17.start
  measures "d184" distance between parallel lines of L16 L2
  measures "d185" distance between parallel lines of L5 L13
  measures "d186" distance of L1.end L2.end
  measures "d187" distance of L11.end L9.start
extrude "Extrusion40" cut sketch "Sketch59" against normal through all
extrude "Extrusion41" cut sketch "Sketch58" against normal blind 132
sketch "Sketch60" plane through (63.8941, 51, 0.081) normal (0, 0, -1) x (-1, 0, 0)
  point P0 (63.8941, -51)
sketch "Sketch61" plane through (0, 51, 0) normal (0, 1, 0) x (1, 0, 0)
  line L0 (-68.1059, -9.581) -> (-68.1059, -0.581) projected
  line L1 (-68.1059, -4.081) -> (63.8941, -4.081)
  line L2 (63.8941, -4.081) -> (63.8941, -3.831)
  line L3 (63.8941, -3.831) -> (-68.1059, -3.831)
  line L4 (-68.1059, -3.831) -> (-68.1059, -4.081)
  line L5 (63.8941, -4.081) -> (-68.1059, -4.081) projected
  line L6 (63.8941, -0.081) -> (63.8941, -4.081) projected
  point P0 (0, 0)
  dimension "d195" = 0.25
  constraints: 8 end point, 2 collinear, 2 parallel, 1 horizontal, 1 perpendicular, 1 point on line
  measures "d195" distance of L1.end L2.end
extrude "Extrusion42" cut sketch "Sketch61" against normal up to surface (25 mm away)
sketch "Sketch63" plane through (63.8941, 26, 9.081) normal (1, 0, 0) x (0, 0, -1)
  circle A0 centre (4, -18.9516) radius 4.5 projected
  circle A1 centre (4, -18.9516) radius 4.6499
  point P0 (9.081, -26)
  constraints: 1 centre point, 1 coincident
extrude "Extrusion43" cut sketch "Sketch63" against normal through all
sketch "Sketch64" plane through (63.8941, 26, 9.081) normal (1, 0, 0) x (0, 0, -1)
  line L0 (0, 0) -> (5.25, 0)
  line L1 (5.25, 0) -> (5.25, -5.777)
  line L2 (5.25, -5.777) -> (0, -5.777)
  line L3 (0, -5.777) -> (0, 0)
  line L4 (5.25, 25) -> (5.25, 0) projected
  point P0 (9.081, -26)
  constraints: 8 end point, 2 parallel, 1 collinear, 1 horizontal, 1 perpendicular
extrude "Extrusion44" cut sketch "Sketch64" against normal through all
sketch "Sketch65" plane through (0, 51, 0) normal (0, 1, 0) x (1, 0, 0)
  point P0 (0, 0)
sketch "Sketch66" plane through (43.8941, 26, 9.081) normal (1, 0, 0) x (0, 0, -1)
  line L0 (0, 0) -> (4.4, 0) projected
  line L1 (5.25, -5.777) -> (0, -5.777) projected
  line L2 (0, 0) -> (4.4, 0)
  line L3 (4.4, 0) -> (4.4, -5.777)
  line L4 (4.4, -5.777) -> (0, -5.777)
  line L5 (0, -5.777) -> (0, 0)
  line L6 (4.4, 0) -> (4.4, 19) projected
  point P0 (9.081, -26)
  constraints: 8 end point, 2 parallel, 1 collinear, 1 horizontal, 1 perpendicular, 1 point on line
sketch "Sketch67" plane through (43.8941, 26, 9.081) normal (1, 0, 0) x (0, 0, -1)
  point P0 (9.081, -26)
sketch "Sketch68" plane through (43.8941, 26, 9.081) normal (1, 0, 0) x (0, 0, -1)
  point P0 (9.081, -26)
extrude "Extrusion45" add sketch "Sketch66" against normal up to surface (1.1 mm away)
sketch "Sketch69" plane through (43.8941, 20.223, 9.081) normal (1, 0, 0) x (0, 0, -1)
  line L0 (0, 0) -> (5.25, 0) projected
  line L1 (4.4, 24.777) -> (0, 24.777)
  line L2 (0, 24.777) -> (0, 0)
  line L3 (0, 0) -> (4.4, 0)
  line L4 (4.4, 0) -> (4.4, 24.777)
  point P0 (9.081, -20.223)
  constraints: 8 end point, 2 parallel, 1 horizontal, 1 perpendicular
extrude "Extrusion46" cut sketch "Sketch69" against normal through all
sketch "Sketch70" plane through (43.8941, 45, 9.081) normal (1, 0, 0) x (0, 0, -1)
  line L0 (0, -24.777) -> (0, 6) projected
  line L1 (0, -24.777) -> (4.4, -24.777)
  line L2 (4.4, -24.777) -> (4.4, -8.0833)
  line L3 (4.4, -8.0833) -> (0, -8.0833)
  line L4 (0, -8.0833) -> (0, -24.777)
  point P0 (9.081, -45)
  constraints: 8 end point, 2 parallel, 1 horizontal, 1 perpendicular
extrude "Extrusion47" add sketch "Sketch70" against normal blind 1.1
pattern_linear "Rectangular Pattern10" count 12 spacing 2.5 along (-1, 0, 0) of "Extrusion47"
sketch "Sketch71" plane through (63.8941, 51, 12.081) normal (1, 0, 0) x (0, 0, -1)
  point P0 (12.081, -51)
sketch "Sketch72" plane through (63.8941, 51, 12.081) normal (1, 0, 0) x (0, 0, -1)
  line L0 (0, 0) -> (3, 0) projected
  line L1 (12, 0) -> (12, -30.9976) projected
  line L2 (0, 0) -> (12, 0)
  line L3 (12, 0) -> (12, -8.7758)
  line L4 (12, -8.7758) -> (0, -8.7758)
  line L5 (0, -8.7758) -> (0, 0)
  point P0 (12.081, -51)
  constraints: 8 end point, 2 parallel, 1 horizontal, 1 perpendicular, 1 point on line
sketch "Sketch73" plane through (-48.1059, 45, 9.081) normal (-1, 0, 0) x (0, 0, 1)
  line L0 (0, -8.0833) -> (-4.4, -8.0833) projected
  line L1 (0, -8.0833) -> (0, -24.777) projected
  line L2 (-4.4, -8.0833) -> (0, -8.0833)
  line L3 (0, -8.0833) -> (0, -24.777)
  line L4 (0, -24.777) -> (-4.4, -24.777)
  line L5 (-4.4, -24.777) -> (-4.4, -8.0833)
  point P0 (-9.081, -45)
  constraints: 8 end point, 2 parallel, 1 horizontal, 1 perpendicular
extrude "Extrusion49" add sketch "Sketch73" against normal blind 1.1
pattern_linear "Rectangular Pattern11" count 12 spacing 2.5 along (1, 0, 0) of "Extrusion49"
extrude "Extrusion50" cut sketch "Sketch72" against normal through all
sketch "Sketch74" plane through (63.8941, 20.223, 9.081) normal (0, 1, 0) x (1, 0, 0)
  line L0 (0, 5.25) -> (-132, 5.25) projected
  line L1 (-110.9, 5.25) -> (-112, 5.25)
  line L2 (-112, 5.25) -> (-112, 0.85)
  line L3 (-112, 0.85) -> (-110.9, 0.85)
  line L4 (-110.9, 0.85) -> (-110.9, 5.25)
  line L5 (-110.9, 4.4) -> (-110.9, 0) projected
  line L6 (-112, 0) -> (-112, 4.4) projected
  point P0 (-63.8941, 9.081)
  dimension "d223" = 4.4
  constraints: 8 end point, 2 collinear, 2 parallel, 1 horizontal, 1 perpendicular, 1 point on line
  measures "d223" distance of L1.end L2.end
sketch "Sketch75" plane through (63.8941, 20.223, 9.081) normal (0, 1, 0) x (1, 0, 0)
  line L0 (0, 5.25) -> (-132, 5.25) projected
  line L1 (-132, 0) -> (0, 0) projected
  line L2 (-82.2249, 5.25) -> (-118.0941, 5.25)
  line L3 (-118.0941, 5.25) -> (-118.0941, 0)
  line L4 (-118.0941, 0) -> (-82.2249, 0)
  line L5 (-82.2249, 0) -> (-82.2249, 5.25)
  point P0 (-63.8941, 9.081)
  constraints: 8 end point, 2 parallel, 2 point on line, 1 horizontal, 1 perpendicular
extrude "Extrusion51" cut sketch "Sketch75" along normal through all
extrude "Extrusion52" add sketch "Sketch74" along normal blind 16.9
pattern_linear "Rectangular Pattern12" count 12 spacing 2.5 along (1, 0, 0) of "Extrusion52"
sketch "Sketch76" plane through (63.8941, 20.223, 9.081) normal (0, 1, 0) x (1, 0, 0)
  line L0 (-48.6, 0) -> (-48.6, 4.4) projected
  line L1 (0, 5.25) -> (-83.4, 5.25) projected
  line L2 (-48.6, 0.85) -> (-47.5, 0.85)
  line L3 (-47.5, 0.85) -> (-47.5, 5.25)
  line L4 (-47.5, 5.25) -> (-48.6, 5.25)
  line L5 (-48.6, 5.25) -> (-48.6, 0.85)
  line L6 (-47.5, 4.4) -> (-47.5, 0) projected
  point P0 (-63.8941, 9.081)
  dimension "d231" = 4.4
  constraints: 8 end point, 2 parallel, 2 point on line, 1 collinear, 1 horizontal, 1 perpendicular
  measures "d231" distance of L4.end L2.start
sketch "Sketch77" plane through (63.8941, 20.223, 9.081) normal (0, 1, 0) x (1, 0, 0)
  line L0 (-19.0354, 0) -> (-51.8906, 0)
  line L1 (-51.8906, 0) -> (-51.8906, 4.9592)
  line L2 (-51.8906, 4.9592) -> (-19.0354, 4.9592)
  line L3 (-19.0354, 4.9592) -> (-19.0354, 0)
  line L4 (-132, 0) -> (0, 0) projected
  point P0 (-63.8941, 9.081)
  constraints: 8 end point, 2 parallel, 1 collinear, 1 horizontal, 1 perpendicular
extrude "Extrusion53" cut sketch "Sketch77" along normal through all
extrude "Extrusion54" add sketch "Sketch76" along normal blind 16.9
pattern_linear "Rectangular Pattern13" count 12 spacing 2.5 along (1, 0, 0) of "Extrusion54"
sketch "Sketch78" plane through (-48.1059, -0.8076, 12.081) normal (0, 0, 1) x (1, 0, 0)
  line L0 (18.6, 16.81) -> (18.6, 2) projected
  line L1 (18.6, 16.81) -> (10.6, 16.81)
  line L2 (10.6, 16.81) -> (10.6, 2)
  line L3 (10.6, 2) -> (18.6, 2)
  line L4 (18.6, 2) -> (18.6, 16.81)
  line L5 (73.4, 2) -> (18.6, 2) projected
  line L6 (73.4, 16.81) -> (81.4, 16.81)
  line L7 (81.4, 16.81) -> (81.4, 2)
  line L8 (81.4, 2) -> (73.4, 2)
  line L9 (73.4, 2) -> (73.4, 16.81)
  line L10 (18.6, 16.81) -> (73.4, 16.81) projected
  line L11 (73.4, 16.81) -> (73.4, 2) projected
  point P0 (48.1059, 0.8076)
  dimension "d239" = 8
  dimension "d240" = 8
  constraints: 16 end point, 4 collinear, 4 parallel, 2 horizontal, 2 perpendicular
  measures "d239" distance of L3.end L2.end
  measures "d240" distance of L7.end L8.end
extrude "Extrusion55" cut sketch "Sketch78" against normal through all contours L0 L3 L2 L1 | L6 L7 L8 L9
sketch "Sketch79" plane through (-48.1059, -0.8076, 12.081) normal (0, 0, 1) x (1, 0, 0)
  line L0 (-20, 20.81) -> (-20, 0) projected
  line L1 (-20, 0) -> (-10, 0)
  line L2 (-10, 0) -> (-10, -5)
  line L3 (-10, -5) -> (-20, -5)
  line L4 (-20, -5) -> (-20, 0)
  line L5 (0, 16.81) -> (0, 0) projected
  line L6 (0, 0) -> (92, 0)
  line L7 (92, 0) -> (92, -5)
  line L8 (92, -5) -> (0, -5)
  line L9 (0, -5) -> (0, 0)
  line L10 (102, 0) -> (112, 0) projected
  line L11 (102, 0) -> (112, 0)
  line L12 (112, 0) -> (112, -5)
  line L13 (112, -5) -> (102, -5)
  line L14 (102, -5) -> (102, 0)
  line L15 (-10, 0) -> (-10, 16.81) projected
  line L16 (92, 0) -> (92, 16.81) projected
  line L17 (112, 43.0318) -> (112, 0) projected
  point P0 (48.1059, 0.8076)
  dimension "d243" = 5
  dimension "d244" = 5
  dimension "d245" = 5
  constraints: 24 end point, 6 parallel, 3 collinear, 3 horizontal, 3 perpendicular
  measures "d243" distance of L1.end L2.end
  measures "d244" distance of L6.end L7.end
  measures "d245" distance of L11.end L12.end
extrude "Extrusion56" add sketch "Sketch79" against normal up to surface (25 mm away)
sketch "Sketch80" plane through (-58.1059, 16.0024, 12.081) normal (0, 0, 1) x (1, 0, 0)
  line L0 (20.6, -14.81) -> (20.6, 0) projected
  line L1 (20.6, -14.81) -> (91.4, -14.81)
  line L2 (91.4, -14.81) -> (91.4, -20.81)
  line L3 (91.4, -20.81) -> (20.6, -20.81)
  line L4 (20.6, -20.81) -> (20.6, -14.81)
  line L5 (91.4, 0) -> (91.4, -14.81) projected
  point P0 (58.1059, -16.0024)
  dimension "d248" = 6
  constraints: 8 end point, 2 parallel, 1 collinear, 1 horizontal, 1 perpendicular
  measures "d248" distance of L1.end L2.end
extrude "Extrusion57" cut sketch "Sketch80" against normal up to next
sketch "Sketch81" plane through (63.8941, 20.0024, 0.081) normal (1, 0, 0) x (0, 0, -1)
  circle A0 centre (-5, -12.954) radius 4.6499 projected
  line L0 (-5, -12.954) -> (-2, -12.954) construction
  line L1 (-2, -12.954) -> (-2, -14.954) construction
  circle A1 centre (-2, -14.954) radius 4.65
  point P0 (0.081, -20.0024)
  dimension "d251" = 3
  dimension "d252" = 2
  dimension "d253" = 9.3
  constraints: 4 end point, 1 centre point, 1 coincident, 1 horizontal, 1 vertical
  measures "d251" distance of L0.start L0.end
  measures "d252" distance of L0.end L1.end
  measures "d253" diameter of A1
sketch "Sketch82" plane through (63.8941, 20.0024, 0.081) normal (1, 0, 0) x (0, 0, -1)
  circle A0 centre (-5, -12.954) radius 4.6499 projected
  circle A1 centre (-5, -12.954) radius 4.6499
  point P0 (0.081, -20.0024)
  constraints: 1 centre point, 1 coincident
extrude "Extrusion58" add sketch "Sketch82" against normal up to surface (132 mm away)
sketch "Sketch83" plane through (-58.1059, 16.0024, 12.081) normal (0, 0, 1) x (1, 0, 0)
  line L0 (0, 0) -> (10, 0) projected
  line L1 (10, -21.81) -> (102, -21.81) projected
  line L2 (0, 0) -> (10, 0)
  line L3 (10, 0) -> (10, -21.81)
  line L4 (10, -21.81) -> (0, -21.81)
  line L5 (0, -21.81) -> (0, 0)
  line L6 (91.4, 0) -> (20.6, 0) projected
  line L7 (91.4, -20.81) -> (91.4, 0) projected
  line L8 (20.6, 0) -> (91.4, 0)
  line L9 (91.4, 0) -> (91.4, -20.81)
  line L10 (91.4, -20.81) -> (20.6, -20.81)
  line L11 (20.6, -20.81) -> (20.6, 0)
  line L12 (102, 0) -> (102, -21.81) projected
  line L13 (102, 0) -> (112, 0)
  line L14 (112, 0) -> (112, -21.81)
  line L15 (112, -21.81) -> (102, -21.81)
  line L16 (102, -21.81) -> (102, 0)
  point P0 (58.1059, -16.0024)
  constraints: 24 end point, 6 parallel, 3 horizontal, 3 perpendicular
extrude "Extrusion59" cut sketch "Sketch83" against normal blind 16.9
extrude "Extrusion60" cut sketch "Sketch81" against normal up to surface (132 mm away) contours A0 A1 | A0 A1 picked at (-4.5196, -13.8416) picked at (0.7979, -16.9283)
draft "FaceDraft14" angle 40 pull direction (0, 0, 1) faces at (43.1608, 37.123, 5.2976) (40.6608, 37.123, 5.2976) (38.1608, 37.123, 5.2976) (35.6608, 37.123, 5.2976) (33.1608, 37.123, 5.2976) (30.6608, 37.123, 5.2976) (28.1608, 37.123, 5.2976) (25.6608, 37.123, 5.2976) (23.1608, 37.123, 5.2976) (20.6608, 37.123, 5.2976) (18.1608, 37.123, 5.2976) (15.6608, 37.123, 5.2976) (-20.2392, 37.123, 5.2976) (-22.7392, 37.123, 5.2976) (-25.2392, 37.123, 5.2976) (-27.7392, 37.123, 5.2976) (-30.2392, 37.123, 5.2976) (-32.7392, 37.123, 5.2976) (-35.2392, 37.123, 5.2976) (-37.7392, 37.123, 5.2976) (-40.2392, 37.123, 5.2976) (-42.7392, 37.123, 5.2976) (-45.2392, 37.123, 5.2976) (-47.7392, 37.123, 5.2976) fixed edges at (43.3441, 37.123, 8.231) (40.8441, 37.123, 8.231) (38.3441, 37.123, 8.231) (35.8441, 37.123, 8.231) (33.3441, 37.123, 8.231) (30.8441, 37.123, 8.231) (28.3441, 37.123, 8.231) (25.8441, 37.123, 8.231) (23.3441, 37.123, 8.231) (20.8441, 37.123, 8.231) (18.3441, 37.123, 8.231) (15.8441, 37.123, 8.231) (-20.0559, 37.123, 8.231) (-22.5559, 37.123, 8.231) (-25.0559, 37.123, 8.231) (-27.5559, 37.123, 8.231) (-30.0559, 37.123, 8.231) (-32.5559, 37.123, 8.231) (-35.0559, 37.123, 8.231) (-37.5559, 37.123, 8.231) (-40.0559, 37.123, 8.231) (-42.5559, 37.123, 8.231) (-45.0559, 37.123, 8.231) (-47.5559, 37.123, 8.231)
sketch "Sketch85" plane through (63.8941, 20.0024, 0.081) normal (1, 0, 0) x (0, 0, -1)
  circle A0 centre (-2, -14.954) radius 4.65 construction
  line L0 (-2, -14.954) -> (-2, -17.954) construction
  circle A1 centre (-2, -17.954) radius 4.7
  point P0 (0.081, -20.0024)
  dimension "d261" = 3
  dimension "d262" = 9.4
  constraints: 2 end point, 1 centre point, 1 coincident, 1 vertical
  measures "d261" distance of L0.start L0.end
  measures "d262" diameter of A1
sketch "Sketch86" plane through (-58.1059, 16.0024, 12.081) normal (0, 0, 1) x (1, 0, 0)
  line L0 (0, 0) -> (10, 0) projected
  line L1 (0, 0) -> (-10, 0)
  line L2 (-10, 0) -> (-10, -23)
  line L3 (-10, -23) -> (0, -23)
  line L4 (0, -23) -> (0, 0)
  line L5 (-10, -21.81) -> (-10, 26.2218) projected
  line L6 (112, 0) -> (102, 0) projected
  line L7 (112, 0) -> (122, 0)
  line L8 (122, 0) -> (122, -23)
  line L9 (122, -23) -> (112, -23)
  line L10 (112, -23) -> (112, 0)
  line L11 (122, 26.2218) -> (122, -21.81) projected
  line L12 (102, 0) -> (91.4, 0)
  line L13 (91.4, 0) -> (91.4, -23)
  line L14 (91.4, -23) -> (102, -23)
  line L15 (102, -23) -> (102, 0)
  line L16 (91.4, 0) -> (91.4, -20.81) projected
  line L17 (10, -21.81) -> (10, 0) projected
  line L18 (10, 0) -> (20.6, 0)
  line L19 (20.6, 0) -> (20.6, -23)
  line L20 (20.6, -23) -> (10, -23)
  line L21 (10, -23) -> (10, 0)
  line L22 (20.6, -20.81) -> (20.6, 0) projected
  point P0 (58.1059, -16.0024)
  dimension "d264" = 23
  constraints: 32 end point, 8 parallel, 7 collinear, 4 horizontal, 4 perpendicular
  measures "d264" distance of L9.end L6.start
extrude "Extrusion61" add sketch "Sketch86" against normal up to surface (25 mm away)
extrude "Extrusion62" cut sketch "Sketch85" against normal up to surface (132 mm away)
sketch "Sketch87" plane through (43.8941, 16.0024, 12.081) normal (0, 0, 1) x (1, 0, 0)
  line L0 (-81.4, -23) -> (-81.4, -21.81) projected
  line L1 (-10.6, -21.81) -> (-10.6, -23) projected
  line L2 (-81.4, -21.81) -> (-10.6, -21.81)
  line L3 (-10.6, -21.81) -> (-10.6, -23)
  line L4 (-10.6, -23) -> (-81.4, -23)
  line L5 (-81.4, -23) -> (-81.4, -21.81)
  point P0 (-43.8941, -16.0024)
  dimension "d271" = 1.19
  constraints: 8 end point, 2 parallel, 1 horizontal, 1 perpendicular
  measures "d271" distance of L1.start L1.end
sketch "Sketch88" plane through (43.8941, 16.0024, 12.081) normal (0, 0, 1) x (1, 0, 0)
  line L0 (-81.4, 0) -> (-81.4, -20.81) projected
  line L1 (-81.4, -20.81) -> (-10.6, -20.81)
  line L2 (-10.6, -20.81) -> (-10.6, -21.81)
  line L3 (-10.6, -21.81) -> (-81.4, -21.81)
  line L4 (-81.4, -21.81) -> (-81.4, -20.81)
  line L5 (-10.6, -21.81) -> (-81.4, -21.81) projected
  point P0 (-43.8941, -16.0024)
  constraints: 8 end point, 2 parallel, 1 collinear, 1 horizontal, 1 perpendicular
extrude "Extrusion63" cut sketch "Sketch88" against normal up to surface (25 mm away)
extrude "Extrusion64" add sketch "Sketch87" against normal up to surface (25 mm away)
sketch "Sketch89" plane through (-68.1059, 20.0024, -12.919) normal (-1, 0, 0) x (0, 0, 1)
  line L0 (0, 0) -> (6, 0)
  line L1 (6, 0) -> (6, -27)
  line L2 (6, -27) -> (0, -27)
  line L3 (0, -27) -> (0, 0)
  line L4 (25, -27) -> (0, -27) projected
  point P0 (12.919, -20.0024)
  dimension "d276" = 6
  constraints: 8 end point, 2 parallel, 1 collinear, 1 horizontal, 1 perpendicular
  measures "d276" distance of L1.end L2.end
extrude "Extrusion65" cut sketch "Sketch89" against normal up to surface (132 mm away)
body "Solid2"
